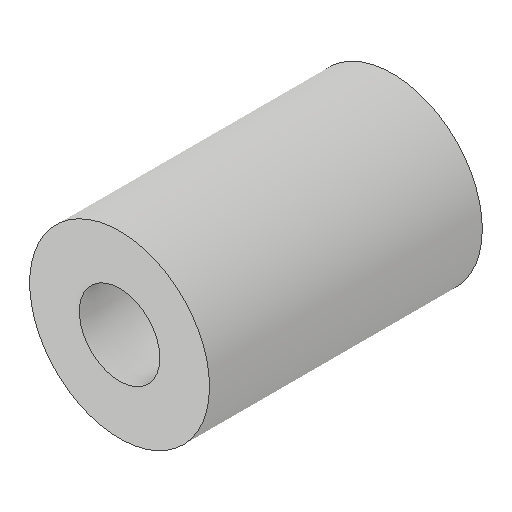
# Autodesk Inventor part: 3DP_PLA_11mm_M3_Standoff
Saved by Autodesk Inventor 2025 (Build 290162010, 162A)
## iProperties
Created: 2019-02-18
Part Number: 3DP_PLA_11mm_M3_Standoff
Material: Generic
Document SubType Name: Modeling
Designer: Andrzej
Density: 1 g/cm^3
Appearance: Default
Author: Andrzej
Autodesk Inventor part; units mm, degrees
ref_plane "YZ Plane" through (0, 0, 0) normal (1, 0, 0) x (0, 1, 0)
ref_plane "XZ Plane" through (0, 0, 0) normal (0, 1, 0) x (-1, 0, 0)
ref_plane "XY Plane" through (0, 0, 0) normal (0, 0, 1) x (1, 0, 0)
sketch "Sketch1" plane through (0, 0, 0) normal (0, 0, 1) x (1, 0, 0)
  circle A0 centre (0, 0) radius 1.625
  circle A1 centre (0, 0) radius 3.625
  dimension "d0" = 3.25
  dimension "d1" = 2
  dimension "d2" = 7.25
  constraints: 2 centre point, 1 coincident
  measures "d0" diameter of A0
  measures "d1" radial gap between concentric circles of A0 A1
  measures "d2" diameter of A1
extrude "Extrusion1" add sketch "Sketch1" along normal blind 11
body "Solid1"
